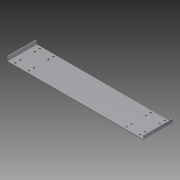
# Autodesk Inventor part: Base Crossbar
Saved by Autodesk Inventor 2012 (Build 160160000, 160)
## iProperties
Created: 2011-10-13
Part Number: Base Crossbar
Material: Default
Document SubType Name: Sheet Metal
Designer: Tushar
Density: 1 g/cm^3
Sheet Metal Rule: Default
Author: Tushar
Autodesk Inventor part; units mm, degrees
ref_plane "YZ Plane" through (0, 0, 0) normal (1, 0, 0) x (0, 1, 0)
ref_plane "XZ Plane" through (0, 0, 0) normal (0, 1, 0) x (-1, 0, 0)
ref_plane "XY Plane" through (0, 0, 0) normal (0, 0, 1) x (1, 0, 0)
sketch "Sketch2" plane through (0, 0, 0) normal (0, 1, 0) x (-1, 0, 0)
  line L0 (-292.481, 63.5) -> (292.481, 63.5)
  line L1 (292.481, 63.5) -> (292.481, -63.5)
  line L2 (292.481, -63.5) -> (-292.481, -63.5)
  line L3 (-292.481, -63.5) -> (-292.481, 63.5)
  point P0 (0, 0)
  dimension "d0" = 292.481
  dimension "d1" = 292.481
  dimension "d2" = 63.5
  dimension "d3" = 63.5
  measures "d0" distance from line of L1 point (0, 0)
  measures "d1" distance from line of point (0, 0) L3
  measures "d2" distance from line of L2 point (0, 0)
  measures "d3" distance from line of L0 point (0, 0)
extrude "Plate1" add sketch "Sketch2" along normal blind 3.048
sketch "Sketch3" plane through (-292.481, 0, 63.5) normal (0, 0, 1) x (1, 0, 0)
  arc A0 (584.962, 0) -> (591.185, 6.223) centre (584.962, 6.223) ccw
  line L0 (584.962, 6.223) -> (591.185, 6.223) construction
  line L1 (584.962, 6.223) -> (584.962, 0) construction
  line L2 (591.185, 6.223) -> (591.185, 19.5834)
  point P0 (584.962, 3.048)
  point P1 (292.481, 0)
  dimension "d5" = 90
  dimension "d6" = 6.223
  dimension "d7" = 6.223
  dimension "d8" = 13.3604
  measures "d5" angle of L1 L0
  measures "d6" radius of A0
  measures "d7" horizontal distance of point (584.962, 3.048) L0.end
  measures "d8" distance of L0.end L2.end
contour flange "Contour Flange1" sketch "Sketch3" thickness 3.048 bend radius 3.048 curves A0 L2 edges at (292.481, 0, 0) running between points at (292.481, 0, -63.5) (292.481, 0, 63.5)
bend "Bend1"
corner "Corner1"
sketch "Sketch4" plane through (-292.481, 0, 63.5) normal (0, 0, 1) x (1, 0, 0)
  arc A0 (-6.223, 6.223) -> (0, 0) centre (0, 6.223) ccw
  line L0 (0, 6.223) -> (-6.223, 6.223) construction
  line L1 (0, 6.223) -> (0, 0) construction
  line L2 (-6.223, 6.223) -> (-6.223, 19.5834)
  point P0 (0, 3.048)
  point P1 (292.481, 0)
  dimension "d18" = 90
  dimension "d19" = 6.223
  dimension "d20" = 6.223
  dimension "d21" = 13.3604
  measures "d18" angle of L0 L1
  measures "d19" radius of A0
  measures "d20" horizontal distance of point (0, 3.048) L0.end
  measures "d21" distance of L0.end L2.end
contour flange "Contour Flange2" sketch "Sketch4" thickness 3.048 bend radius 3.048 curves A0 L2 edges at (-292.481, 0, 0) running between points at (-292.481, 0, 63.5) (-292.481, 0, -63.5)
bend "Bend2"
corner "Corner2"
sketch "Sketch5" plane through (298.704, 6.223, -63.5) normal (1, 0, 0) x (0, 0, -1)
  line L0 (-127, 0) -> (-127, 13.3604) projected
  line L1 (0, -6.223) -> (-127, -6.223) projected
  point P0 (-63.5, -6.223)
  point P1 (-114.3, 6.477)
  dimension "d31" = 12.7
  dimension "d32" = 12.7
  measures "d31" distance from line of L1 point (-114.3, 6.477)
  measures "d32" distance from line of L0 point (-114.3, 6.477)
hole "Hole1" at (298.704, 12.7, 50.8) direction (-1, 0, 0) diameter 3.175 end through all
sketch "Sketch6" plane through (298.704, 6.223, -63.5) normal (1, 0, 0) x (0, 0, -1)
  circle A0 centre (-114.3, 6.477) radius 1.5875 projected
  line L0 (-127, 0) -> (-127, 13.3604) projected
  line L1 (-114.3, 6.477) -> (-99.9256, 6.477)
  point P0 (-63.5, -6.223)
  constraints: 2 end point, 1 perpendicular
pattern_linear "Rectangular Pattern1" count 9 spacing 12.7 along (0, 0, -1) of "Hole1"
sketch "Sketch7" plane through (0, 3.048, 0) normal (0, 1, 0) x (1, 0, 0)
  line L0 (292.481, -63.5) -> (-292.481, -63.5) projected
  line L1 (-292.481, 63.5) -> (292.481, 63.5) projected
  line L2 (298.704, 63.5) -> (298.704, -63.5) projected
  line L3 (-298.704, -63.5) -> (-298.704, 63.5) projected
  point P0 (0, 0)
  point P1 (272.0086, -53.34)
  point P2 (272.0086, 53.34)
  point P3 (-272.0086, -53.34)
  point P4 (-272.0086, 53.34)
  point P5 (-272.0086, 31.3944)
  point P6 (-272.0086, -31.3944)
  point P7 (272.0086, -31.3944)
  point P8 (272.0086, 31.3944)
  point P9 (-212.725, -53.34)
  point P10 (-212.725, -31.3944)
  point P11 (-212.725, 31.3944)
  point P12 (-212.725, 53.34)
  point P13 (212.725, -53.34)
  point P14 (212.725, -31.3944)
  point P15 (212.725, 31.3944)
  point P16 (212.725, 53.34)
  dimension "d43" = 26.6954
  dimension "d44" = 10.16
  dimension "d45" = 10.16
  dimension "d46" = 26.6954
  dimension "d54" = 84.7344
  dimension "d55" = 84.7344
  dimension "d56" = 59.2836
  dimension "d57" = 59.2836
  constraints: 12 horizontal alignment, 12 vertical alignment
  measures "d43" distance from line of L2 point (272.009, -53.34)
  measures "d44" distance from line of L0 point (272.009, -53.34)
  measures "d45" distance from line of L1 point (272.009, 53.34)
  measures "d46" distance from line of L3 point (-272.009, -53.34)
  measures "d54" distance of point (-272.009, -53.34) point (-272.009, 31.394)
  measures "d55" distance of point (-272.009, -31.394) point (-272.009, 53.34)
  measures "d56" distance of point (-212.725, -53.34) point (-272.009, -53.34)
  measures "d57" distance of point (212.725, -53.34) point (272.009, -53.34)
hole "Hole3" at (272.0086, 3.048, 53.34) at (272.0086, 3.048, -53.34) at (-272.0086, 3.048, 53.34) at (-272.0086, 3.048, -53.34) at (-272.0086, 3.048, -31.3944) at (-272.0086, 3.048, 31.3944) at (272.0086, 3.048, 31.3944) at (272.0086, 3.048, -31.3944) at (-212.725, 3.048, 53.34) at (-212.725, 3.048, 31.3944) at (-212.725, 3.048, -31.3944) at (-212.725, 3.048, -53.34) at (212.725, 3.048, 53.34) at (212.725, 3.048, 31.3944) at (212.725, 3.048, -31.3944) at (212.725, 3.048, -53.34) direction (0, -1, 0) diameter 8.382 end through all
equation "\"d38\" = Thickness"
equation "\"d63\" = Thickness"
equation "\"d9\" = BendReliefWidth"
equation "\"d10\" = BendReliefDepth"
equation "\"d11\" = MinimumRemnant"
equation "\"d12\" = BendRadius"
equation "\"d13\" = BendRadius"
equation "\"d15\" = CornerReliefSize"
equation "\"d16\" = GapSize"
equation "\"d17\" = JacobiRadiusSize"
equation "\"d22\" = BendReliefWidth"
equation "\"d23\" = BendReliefDepth"
equation "\"d24\" = MinimumRemnant"
equation "\"d25\" = BendRadius"
equation "\"d26\" = BendRadius"
equation "\"d28\" = CornerReliefSize"
equation "\"d29\" = GapSize"
equation "\"d30\" = JacobiRadiusSize"
equation "\"d1\" = d0"
equation "\"d3\" = d2"
equation "\"BendRadius\" = Thickness"
equation "\"BendReliefWidth\" = Thickness"
equation "\"BendReliefDepth\" = 0.5 * Thickness"
equation "\"CornerReliefSize\" = 4 * Thickness"
equation "\"MinimumRemnant\" = 2 * Thickness"
equation "\"TransitionRadius\" = BendRadius"
equation "\"JacobiRadiusSize\" = BendRadius"
equation "\"GapSize\" = Thickness"
equation "\"d4\" = BendRadius"
equation "\"Thickness\" = 3.048"
body "Solid1"
